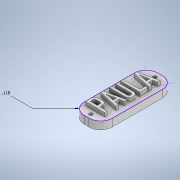
# Autodesk Inventor part: temp1
Saved by Autodesk Inventor 2021 (Build 250183000, 183)
## iProperties
Created: 2023-12-10
Part Number: temp1
Material: Generic
Document SubType Name: Modeling
Designer: assman
Density: 1 g/cm^3
Appearance: Default
Author: assman
## iProperties of the stored document _3DPrint.ipt
Created: 2023-12-10
Part Number: _3DPrint
Material: Generic
Document SubType Name: Modeling
Designer: assman
Density: 1 g/cm^3
Appearance: Default
Author: assman
Autodesk Inventor part; units mm, degrees
ref_plane "YZ Plane" through (0, 0, 0) normal (1, 0, 0) x (0, 1, 0)
ref_plane "XZ Plane" through (0, 0, 0) normal (0, 1, 0) x (-1, 0, 0)
ref_plane "XY Plane" through (0, 0, 0) normal (0, 0, 1) x (1, 0, 0)
sketch "Sketch1" plane through (0, 0, 0) normal (0, 1, 0) x (-1, 0, 0)
  line L0 (0.6121, 9.4217) -> (-0.6121, 9.4217)
  line L1 (-3.6121, 6.4217) -> (-3.6121, -6.4217)
  line L2 (-0.6121, -9.4217) -> (0.6121, -9.4217)
  line L3 (3.6121, -6.4217) -> (3.6121, 6.4217)
  line L4 (3.6121, 9.4217) -> (-3.6121, -9.4217) construction
  line L5 (-3.6121, 9.4217) -> (3.6121, -9.4217) construction
  arc A0 (3.6121, 6.4217) -> (0.6121, 9.4217) centre (0.6121, 6.4217) ccw
  arc A1 (-0.6121, 9.4217) -> (-3.6121, 6.4217) centre (-0.6121, 6.4217) ccw
  arc A2 (0.6121, -9.4217) -> (3.6121, -6.4217) centre (0.6121, -6.4217) ccw
  arc A3 (-3.6121, -6.4217) -> (-0.6121, -9.4217) centre (-0.6121, -6.4217) ccw
  line L6 (2.5462, 7.5291) -> (2.5462, -7.1828) construction
  line L7 (2.5462, -7.1828) -> (-2.4754, -7.1828) construction
  line L8 (-2.4754, -7.1828) -> (-2.4754, 7.5291) construction
  line L9 (-2.4754, 7.5291) -> (2.5462, 7.5291) construction
  line L10 (0.1215, 6.8275) -> (0.1215, 5.888)
  spline S0 degree 2 poles (0.1215, 5.888) (0.1215, 5.7568) (0.2446, 5.5598) (0.4744, 5.4573) (0.6385, 5.4573) knots 0 0 0 1 2 3 3 3
  line L11 (0.6385, 5.4573) -> (1.3974, 5.4573)
  spline S1 degree 2 poles (1.3974, 5.4573) (1.5656, 5.4573) (1.8036, 5.5598) (1.9308, 5.7568) (1.9308, 5.888) knots 0 0 0 1 2 3 3 3
  line L12 (1.9308, 5.888) -> (1.9308, 6.8275)
  line L13 (1.9308, 6.8275) -> (2.5462, 6.8275)
  line L14 (2.5462, 6.8275) -> (2.5462, 5.9004)
  spline S2 degree 2 poles (2.5462, 5.9004) (2.5462, 5.5516) (2.2795, 5.0552) (1.7667, 4.7968) (1.4097, 4.7968) knots 0 0 0 1 2 3 3 3
  line L15 (1.4097, 4.7968) -> (0.6179, 4.7968)
  spline S3 degree 2 poles (0.6179, 4.7968) (0.2692, 4.7968) (-0.2313, 5.0593) (-0.4939, 5.5557) (-0.4939, 5.9004) knots 0 0 0 1 2 3 3 3
  line L16 (-0.4939, 5.9004) -> (-0.4939, 6.8275)
  line L17 (-0.4939, 6.8275) -> (0.1215, 6.8275)
  line L18 (2.5462, 7.1886) -> (2.5462, 6.5363)
  line L19 (2.5462, 6.5363) -> (-2.4221, 6.5363)
  line L20 (-2.4221, 6.5363) -> (-2.4221, 7.1886)
  line L21 (-2.4221, 7.1886) -> (2.5462, 7.1886)
  line L22 (2.5462, 3.2173) -> (2.5462, 2.6224)
  line L23 (2.5462, 2.6224) -> (-2.4221, 1.4737)
  line L24 (-2.4221, 1.4737) -> (-2.4221, 2.1711)
  line L25 (-2.4221, 2.1711) -> (1.5287, 2.9219)
  line L26 (1.5287, 2.9219) -> (-2.4221, 3.6685)
  line L27 (-2.4221, 3.6685) -> (-2.4221, 4.366)
  line L28 (-2.4221, 4.366) -> (2.5462, 3.2173)
  line L29 (-0.7277, 3.6316) -> (-0.7277, 2.1588)
  line L30 (-0.7277, 2.1588) -> (-1.339, 2.1588)
  line L31 (-1.339, 2.1588) -> (-1.339, 3.6316)
  line L32 (-1.339, 3.6316) -> (-0.7277, 3.6316)
  spline S4 degree 2 poles (-2.4713, -0.0648) (-2.4713, 0.2962) (-2.2046, 0.8049) (-1.6795, 1.0634) (-1.3062, 1.0634) knots 0 0 0 1 2 3 3 3
  line L33 (-1.3062, 1.0634) -> (2.5462, 1.0634)
  line L34 (2.5462, 1.0634) -> (2.5462, 0.4152)
  line L35 (2.5462, 0.4152) -> (-1.3308, 0.4152)
  spline S5 degree 2 poles (-1.3308, 0.4152) (-1.5769, 0.4152) (-1.8395, 0.169) (-1.8395, -0.0648) knots 0 0 0 1 2 2 2
  spline S6 degree 2 poles (-1.8395, -0.0648) (-1.8395, -0.2987) (-1.5769, -0.5489) (-1.3308, -0.5489) knots 0 0 0 1 2 2 2
  line L36 (-1.3308, -0.5489) -> (2.5462, -0.5489)
  line L37 (2.5462, -0.5489) -> (2.5462, -1.1971)
  line L38 (2.5462, -1.1971) -> (-1.3062, -1.1971)
  spline S7 degree 2 poles (-1.3062, -1.1971) (-1.6795, -1.1971) (-2.2046, -0.9346) (-2.4713, -0.4299) (-2.4713, -0.0648) knots 0 0 0 1 2 3 3 3
  line L39 (2.5462, -1.8494) -> (2.5462, -2.5018)
  line L40 (2.5462, -2.5018) -> (-2.4221, -2.5018)
  line L41 (-2.4221, -2.5018) -> (-2.4221, -1.8494)
  line L42 (-2.4221, -1.8494) -> (2.5462, -1.8494)
  line L43 (-1.8067, -2.1982) -> (-1.8067, -3.913)
  line L44 (-1.8067, -3.913) -> (-2.4221, -3.913)
  line L45 (-2.4221, -3.913) -> (-2.4221, -2.1982)
  line L46 (-2.4221, -2.1982) -> (-1.8067, -2.1982)
  line L47 (2.5462, -5.3366) -> (2.5462, -5.9315)
  line L48 (2.5462, -5.9315) -> (-2.4221, -7.0802)
  line L49 (-2.4221, -7.0802) -> (-2.4221, -6.3828)
  line L50 (-2.4221, -6.3828) -> (1.5287, -5.632)
  line L51 (1.5287, -5.632) -> (-2.4221, -4.8854)
  line L52 (-2.4221, -4.8854) -> (-2.4221, -4.1879)
  line L53 (-2.4221, -4.1879) -> (2.5462, -5.3366)
  line L54 (-0.7277, -4.9223) -> (-0.7277, -6.3951)
  line L55 (-0.7277, -6.3951) -> (-1.339, -6.3951)
  line L56 (-1.339, -6.3951) -> (-1.339, -4.9223)
  line L57 (-1.339, -4.9223) -> (-0.7277, -4.9223)
  point P0 (0, 0)
  dimension "d0" = 3
  constraints: 12 end point, 8 point on circle, 8 point on line, 8 tangent, 4 centre point, 3 equal radius, 2 midpoint, 2 parallel, 1 horizontal, 1 perpendicular, 2 other
  measures "d0" radius of A0
extrude "Extrusion1" add sketch "Sketch1" against normal blind 2 contours A0 L3 A2 L2 A3 L1 A1 L0 | L17 L16 L19 L20 L21 L18 L13 L12 L10 | L10 L19 L16 L17 | L19 L12 S1 L11 S0 L10 | L10 S0 L11 S1 L12 L19 L14 S2 L15 S3 L16 | L12 L13 L14 L19 | L22 L23 L24 L25 L31 L30 L29 L26 L32 L27 L28 | L31 L32 L29 L26 | L26 L29 L25 L31 | L25 L29 L30 L31 | L26 L25 L29 | S4 L33 L34 L35 S5 S6 L36 L37 L38 S7 | L39 L40 L43 L46 L41 L42 | L43 L44 L45 L40 | L40 L41 L46 L43 | L47 L48 L49 L50 L56 L55 L54 L51 L57 L52 L53 | L56 L57 L54 L51 | L51 L54 L50 L56 | L50 L54 L55 L56 | L51 L50 L54
extrude "Extrusion2" add sketch "Sketch1" along normal blind 1 contours L17 L16 L19 L20 L21 L18 L13 L12 L10 | L10 L19 L16 L17 | L10 S0 L11 S1 L12 L19 L14 S2 L15 S3 L16 | L12 L13 L14 L19 | L22 L23 L24 L25 L31 L30 L29 L26 L32 L27 L28 | L31 L32 L29 L26 | L26 L29 L25 L31 | L25 L29 L30 L31 | S4 L33 L34 L35 S5 S6 L36 L37 L38 S7 | L39 L40 L43 L46 L41 L42 | L43 L44 L45 L40 | L40 L41 L46 L43 | L47 L48 L49 L50 L56 L55 L54 L51 L57 L52 L53 | L56 L57 L54 L51 | L51 L54 L50 L56 | L50 L54 L55 L56
sketch "Sketch2" plane through (0, 0, 0) normal (0, 1, 0) x (1, 0, 0)
  circle A0 centre (0, -8.337) radius 0.4289
  circle A1 centre (0, 8.1055) radius 0.4428
  point P0 (0, 0)
  constraints: 2 centre point
extrude "Extrusion3" cut sketch "Sketch2" against normal through all
body "Solid1"
